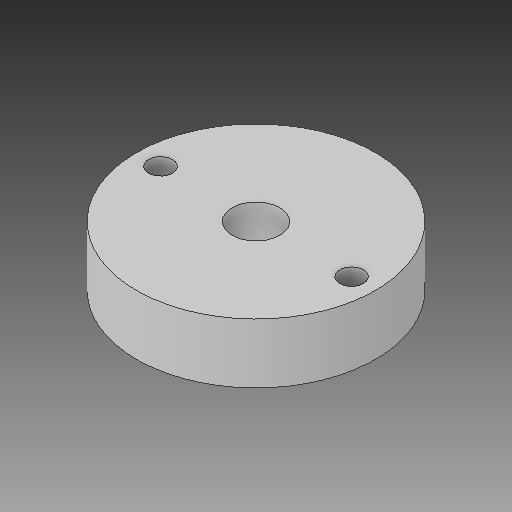
# Autodesk Inventor part: ServoDisk
Saved by Autodesk Inventor 2019 (Build 230136000, 136)
## iProperties
Created: 2019-09-29
Part Number: ServoDisk
Material: Generic
Document SubType Name: Modeling
Designer: james
Density: 1 g/cm^3
Appearance: Default
Mass: 3.02454 g
Surface Area: 16.62 cm^2
Volume: 3.02454 cm^3
Author: james
Autodesk Inventor part; units mm, degrees
ref_plane "YZ Plane" through (0, 0, 0) normal (1, 0, 0) x (0, 1, 0)
ref_plane "XZ Plane" through (0, 0, 0) normal (0, 1, 0) x (-1, 0, 0)
ref_plane "XY Plane" through (0, 0, 0) normal (0, 0, 1) x (1, 0, 0)
sketch "Sketch1" plane through (0, 0, 0) normal (0, 1, 0) x (-1, 0, 0)
  circle A0 centre (0, 0) radius 12.7
  dimension "d0" = 25.4
  constraints: 1 centre point, 1 coincident
  measures "d0" diameter of A0
extrude "Extrusion1" add sketch "Sketch1" along normal blind 6.35
sketch "Sketch2" plane through (0, 6.35, 0) normal (0, 1, 0) x (1, 0, 0)
  circle A0 centre (0, 0) radius 2.54
  circle A1 centre (-10.16, 0) radius 1.27
  circle A2 centre (10.16, 0) radius 1.27
  dimension "d3" = 5.08
  dimension "d4" = 2.54
  dimension "d5" = 2.54
  dimension "d6" = 10.16
  dimension "d7" = 10.16
  constraints: 3 centre point, 1 coincident
  measures "d3" diameter of A0
  measures "d4" diameter of A1
  measures "d5" diameter of A2
  measures "d6" distance of point (0, 0) A1.centre
  measures "d7" distance of A2.centre point (0, 0)
extrude "Extrusion2" cut sketch "Sketch2" against normal blind 6.35
body "Solid1"
